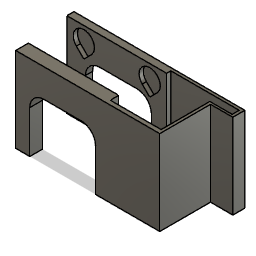
DirtLab_Door_Latch_Holder (Autodesk Fusion 360 design; units mm, degrees)
Autodesk Fusion 360 part; units mm, degrees
sketch "Sketch1" plane through (0, 0, 0) normal (0, 0, 1) x (1, 0, 0)
  line L0 (50, 25) -> (-50, 25)
  line L1 (-50, 25) -> (-50, -25)
  line L2 (-50, -25) -> (50, -25)
  line L3 (50, -25) -> (50, 25)
  line L4 (50, 25) -> (-50, -25) construction
  line L5 (-50, 25) -> (50, -25) construction
  line L6 (-40, -25) -> (6.5, -25) construction
  line L7 (6.5, -25) -> (6.5, 5)
  line L8 (-3.5, 15) -> (-30, 15)
  line L9 (-40, 5) -> (-40, -25)
  arc A0 (-30, 15) -> (-40, 5) centre (-30, 5) ccw
  arc A1 (6.5, 5) -> (-3.5, 15) centre (-3.5, 5) ccw
  line L10 (50, 25) -> (52, 25)
  line L11 (52, 25) -> (52, -25)
  line L12 (52, -25) -> (50, -25)
  line L13 (50, -25) -> (50, 25)
  line L14 (50, 25) -> (14, 25)
  line L15 (14, 25) -> (14, -25)
  line L16 (14, -25) -> (50, -25)
  line L17 (50, -25) -> (50, 25)
  point P0 (-40, 15)
  dimension "d12" = 100
  dimension "d13" = 50
  dimension "d14" = 46.5
  dimension "d15" = 40
  dimension "d16" = 10
  dimension "d17" = 10
  dimension "d18" = 10
  dimension "d19" = 2
  dimension "d20" = 36
  constraint horizontal L0
  constraint perpendicular L0 L1
  constraint parallel L0 L2
  constraint parallel L1 L3
  constraint coincident L4 origin
  constraint coincident L5 origin
  constraint horizontal L6
  constraint vertical L7
  constraint horizontal L8
  constraint vertical L9
  constraint coincident L2 L6.start
  constraint coincident P0 L9
  constraint coincident P0 L8
  constraint tangent L9 A0
  constraint tangent L8 A0
  constraint tangent L8 A1
  constraint tangent L7 A1
  constraint horizontal L10
  constraint vertical L11
  constraint horizontal L12
  constraint vertical L13
  constraint horizontal L14
  constraint vertical L15
  constraint horizontal L16
  constraint vertical L17
  measures "d12" distance of L1.end L2.end
  measures "d13" distance of L0.end L1.end
  measures "d14" distance of L6.start L6.end
  measures "d15" distance of L6.start P0
  measures "d16" distance of L1 L9
  measures "d17" radius of A0
  measures "d18" radius of A1
  measures "d19" distance of L0.start L10.end
  measures "d20" distance of L0.start L14.end
extrude "Extrude1" add sketch "Sketch1" against normal blind 3 contours L0 L2 L3 L13 L14 L15 L16 L17
extrude "Extrude2" add sketch "Sketch1" against normal blind 9 contours L0 L1 L2 L7 L8 L9 A0 A1 L15
extrude "Extrude3" add sketch "Sketch1" against normal blind 37.45 contours L3 L10 L11 L12 L13 L17
sketch "Sketch2" plane through (52, 0, 0) normal (1, 0, 0) x (0, 0, -1)
  line L0 (0, 25) -> (0, -25)
  line L1 (0, -25) -> (37.45, -25)
  line L2 (37.45, -25) -> (37.45, 25)
  line L3 (37.45, 25) -> (0, 25)
  line L4 (37.45, 25) -> (35.95, 25)
  line L5 (35.95, 25) -> (35.95, -25)
  line L6 (35.95, -25) -> (37.45, -25)
  line L7 (37.45, -25) -> (37.45, 25)
  dimension "d27" = 1.5
  constraint horizontal L4
  constraint vertical L5
  constraint horizontal L6
  constraint vertical L7
  constraint coincident L2.end L3.start
  measures "d27" distance of L2.end L4.end
extrude "Extrude4" add sketch "Sketch2" along normal blind 15.8 contours L1 L2 L3 L4 L5 L6 L7
sketch "Sketch3" plane through (0, 0, -37.45) normal (0, 0, -1) x (-1, 0, 0)
  line L0 (-67.8, -25) -> (-50, -25)
  line L1 (-50, -25) -> (-50, 25)
  line L2 (-50, 25) -> (-67.8, 25)
  line L3 (-67.8, 25) -> (-67.8, -25)
  line L4 (-67.8, 25) -> (-65.8, 25)
  line L5 (-65.8, 25) -> (-65.8, -25)
  line L6 (-65.8, -25) -> (-67.8, -25)
  line L7 (-67.8, -25) -> (-67.8, 25)
  dimension "d30" = 2
  constraint horizontal L4
  constraint vertical L5
  constraint horizontal L6
  constraint vertical L7
  constraint coincident L2.end L3.start
  measures "d30" distance of L2.end L4.end
extrude "Extrude5" add sketch "Sketch3" along normal blind 7 contours L0 L2 L3 L4 L5 L6 L7
sketch "Sketch4" plane through (65.8, 0, 0) normal (-1, 0, 0) x (0, 0, 1)
  line L0 (-37.45, -25) -> (-37.45, 25)
  line L1 (-37.45, 25) -> (-44.45, 25)
  line L2 (-44.45, 25) -> (-44.45, -25)
  line L3 (-44.45, -25) -> (-37.45, -25)
  line L4 (-44.45, 25) -> (-42.45, 25)
  line L5 (-42.45, 25) -> (-42.45, -25)
  line L6 (-42.45, -25) -> (-44.45, -25)
  line L7 (-44.45, -25) -> (-44.45, 25)
  dimension "d33" = 2
  constraint horizontal L4
  constraint vertical L5
  constraint horizontal L6
  constraint vertical L7
  constraint coincident L1.end L2.start
  measures "d33" distance of L1.end L4.end
extrude "Extrude6" add sketch "Sketch4" along normal blind 104 contours L1 L2 L3 L4 L5 L6 L7
extrude "Extrude7" add 1 faces at (-38.2, -8.3333, -43.1167) along direction (-1, 0, 0) blind 15
extrude "Extrude8" cut sketch "Sketch1" against normal blind 50 contours L2 L7 L8 L9 A0 A1
sketch "Sketch5" plane through (0, 0, -42.45) normal (0, 0, 1) x (1, 0, 0)
  line L0 (-40, -25) -> (-40, 5)
  arc A0 (-30, 15) -> (-40, 5) centre (-30, 5) ccw
  line L1 (-30, 15) -> (-3.5, 15)
  arc A1 (6.5, 5) -> (-3.5, 15) centre (-3.5, 5) ccw
  line L2 (6.5, 5) -> (6.5, -25)
  line L3 (6.5, -25) -> (65.8, -25)
  line L4 (65.8, -25) -> (65.8, 25)
  line L5 (65.8, 25) -> (-53.2, 25)
  line L6 (-53.2, 25) -> (-53.2, -25)
  line L7 (-53.2, -25) -> (-40, -25)
  line L8 (17.4308, 25) -> (17.4308, -25)
  constraint coincident L5 L8.start
  constraint coincident L3 L8.end
  constraint perpendicular L3 L8
extrude "Extrude9" add sketch "Sketch5" along normal blind 3 contours L0 A0 L1 A1 L2 L3 L5 L6 L7 L8
move_face "OffsetFaces1" offset 10 1 faces at (-28.6667, 25, -4)
sketch "Sketch6" plane through (0, 0, -9) normal (0, 0, -1) x (-1, 0, 0)
  line L0 (50, -25) -> (50, 35)
  line L1 (-14, 35) -> (-14, -25)
  line L2 (-14, -25) -> (-6.5, -25)
  line L3 (-6.5, -25) -> (-6.5, 5)
  arc A0 (3.5, 15) -> (-6.5, 5) centre (3.5, 5) ccw
  line L4 (3.5, 15) -> (30, 15)
  arc A1 (40, 5) -> (30, 15) centre (30, 5) ccw
  line L5 (40, 5) -> (40, -25)
  line L6 (40, -25) -> (50, -25)
  line L7 (50, 35) -> (-14, 35)
  line L8 (1.3033, 19.6967) -> (-4, 14.3934)
  line L9 (1.3033, 19.6967) -> (9.9345, 19.6967) construction
  line L10 (-9.3033, 19.6967) -> (-4, 14.3934)
  line L11 (-9.3033, 19.6967) -> (0.614, 19.6967) construction
  line L12 (45.3033, 19.6967) -> (40, 14.3934)
  line L13 (45.3033, 19.6967) -> (55.2304, 19.6967) construction
  line L14 (34.6967, 19.6967) -> (40, 14.3934)
  line L15 (34.6967, 19.6967) -> (44.4675, 19.6967) construction
  arc A2 (45.3033, 19.6967) -> (34.6967, 19.6967) centre (40, 25) ccw
  arc A3 (1.3033, 19.6967) -> (-9.3033, 19.6967) centre (-4, 25) ccw
  dimension "d53" = 15
  dimension "d54" = 10
  dimension "d55" = 10
  dimension "d56" = 15
  dimension "d57" = 10
  dimension "d58" = 10
  dimension "d59" = 135
  dimension "d60" = 45
  dimension "d62" = 135
  dimension "d64" = 45
  constraint horizontal L9
  constraint tangent L8 A3
  constraint horizontal L11
  constraint tangent L10 A3
  constraint horizontal L13
  constraint tangent L12 A2
  constraint horizontal L15
  constraint tangent L14 A2
  measures "d53" diameter of A3
  measures "d54" distance of L7 A3.centre
  measures "d55" distance of L1 A3.centre
  measures "d56" diameter of A2
  measures "d57" distance of L7 A2.centre
  measures "d58" distance of L0 A2.centre
  measures "d59" angle of L8 L9
  measures "d60" angle of L10 L11
  measures "d62" angle of L12 L13
  measures "d64" angle of L14 L15
extrude "Extrude13" cut sketch "Sketch6" against normal blind 3 contours L8 L10 A3 | L12 L14 A2
sketch "Sketch8" plane through (0, 0, -39.45) normal (0, 0, 1) x (1, 0, 0)
  line L0 (-53.2, 35) -> (-53.2, -25)
  line L1 (-53.2, -25) -> (-40, -25)
  line L2 (-40, -25) -> (-40, 5)
  arc A0 (-30, 15) -> (-40, 5) centre (-30, 5) ccw
  line L3 (-30, 15) -> (-3.5, 15)
  arc A1 (6.5, 5) -> (-3.5, 15) centre (-3.5, 5) ccw
  line L4 (6.5, 5) -> (6.5, -25)
  line L5 (6.5, -25) -> (17.4308, -25)
  line L6 (17.4308, -25) -> (17.4308, 35)
  line L7 (17.4308, 35) -> (-53.2, 35)
  line L8 (10.7341, 19.6967) -> (5.4308, 14.3934)
  line L9 (10.7341, 19.6967) -> (20.8, 19.6967) construction
  line L10 (0.1275, 19.6967) -> (5.4308, 14.3934)
  line L11 (0.1275, 19.6967) -> (9.7626, 19.6967) construction
  arc A2 (10.7341, 19.6967) -> (0.1275, 19.6967) centre (5.4308, 25) ccw
  line L12 (-35.8967, 19.6967) -> (-41.2, 14.3934)
  line L13 (-35.8967, 19.6967) -> (-25.7939, 19.6967) construction
  line L14 (-46.5033, 19.6967) -> (-41.2, 14.3934)
  line L15 (-46.5033, 19.6967) -> (-36.1274, 19.6967) construction
  arc A3 (-35.8967, 19.6967) -> (-46.5033, 19.6967) centre (-41.2, 25) ccw
  dimension "d68" = 15
  dimension "d69" = 15
  dimension "d70" = 10
  dimension "d71" = 10
  dimension "d72" = 12
  dimension "d73" = 12
  dimension "d74" = 135
  dimension "d76" = 45
  dimension "d78" = 135
  dimension "d80" = 45
  constraint horizontal L9
  constraint horizontal L11
  constraint tangent L10 A2
  constraint tangent L8 A2
  constraint horizontal L13
  constraint horizontal L15
  constraint tangent L12 A3
  constraint tangent L14 A3
  measures "d68" diameter of A2
  measures "d69" diameter of A3
  measures "d70" distance of L7 A2.centre
  measures "d71" distance of L7 A3.centre
  measures "d72" distance of L0 A3.centre
  measures "d73" distance of L6 A2.centre
  measures "d74" angle of L8 L9
  measures "d76" angle of L10 L11
  measures "d78" angle of L12 L13
  measures "d80" angle of L14 L15
extrude "Extrude14" cut sketch "Sketch8" against normal blind 3 contours L8 L10 A2 | L12 L14 A3
sketch "Sketch7" plane through (0, 0, -39.45) normal (0, 0, 1) x (1, 0, 0)
  line L0 (-53.2, 31) -> (-53.2, -25)
  line L1 (-53.2, -25) -> (-40, -25)
  line L2 (-40, -25) -> (-40, 5)
  arc A0 (-30, 15) -> (-40, 5) centre (-30, 5) ccw
  line L3 (-30, 15) -> (-3.5, 15)
  arc A1 (6.5, 5) -> (-3.5, 15) centre (-3.5, 5) ccw
  line L4 (6.5, 5) -> (6.5, -25)
  line L5 (6.5, -25) -> (17.4308, -25)
  line L6 (17.4308, 31) -> (-53.2, 31)
  circle A2 centre (8, 20) radius 7.5
  circle A3 centre (-44, 20) radius 7.5
  line L7 (17.4308, -25) -> (17.4308, 25)
  line L8 (17.4308, 25) -> (17.4308, 31)
  dimension "d48" = 15
  dimension "d49" = 15
  measures "d48" diameter of A2
  measures "d49" diameter of A3
equation "frame_interface = 35.45 mm"
equation "closing_flap = 15.8 mm"
equation "inside_bulge = 36 mm"
equation "outside_buldge = 47 mm"
equation "closing_flap_thickness = 5 mm"
equation "inside_interface_handle = 90 mm"
equation "inside_bulge_thickness = 9 mm"
equation "inside_handle = 46.5 mm"
equation "outside_bulge_thickness = 4 mm"
equation "outside_interface_handle = 104 mm"
equation "outside_handle = 46.5 mm"
equation "d12 = inside_interface_handle + 10 mm"
equation "d14 = inside_handle"
equation "d20 = inside_bulge"
equation "d25 = -frame_interface - 2 mm"
equation "d28 = closing_flap"
equation "d31 = closing_flap_thickness + 2 mm"
equation "d34 = outside_interface_handle"
